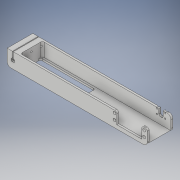
# Autodesk Inventor part: ArmProto1.2
Saved by Autodesk Inventor 2017 (Build 210142000, 142)
## iProperties
Created: 2017-09-30
Part Number: ArmProto1.2
Material: Generic
Document SubType Name: Modeling
Designer: User
Density: 1 g/cm^3
Appearance: Default
Author: User
Autodesk Inventor part; units mm, degrees
ref_plane "YZ Plane" through (0, 0, 0) normal (1, 0, 0) x (0, 1, 0)
ref_plane "XZ Plane" through (0, 0, 0) normal (0, 1, 0) x (-1, 0, 0)
ref_plane "XY Plane" through (0, 0, 0) normal (0, 0, 1) x (1, 0, 0)
sketch "Sketch1" plane through (0, 0, 0) normal (1, 0, 0) x (0, 1, 0)
  line L0 (0, 0) -> (25.4, 0)
  line L1 (25.4, 0) -> (25.4, -42.799)
  line L2 (25.4, -42.799) -> (0, -42.799)
  line L3 (0, -42.799) -> (0, 0)
  line L4 (25.4, -3.175) -> (3.175, -3.175)
  line L5 (3.175, -3.175) -> (3.175, -39.624)
  line L6 (3.175, -39.624) -> (25.4, -39.624)
  line L7 (25.4, -39.624) -> (25.4, -3.175)
  dimension "d0" = 25.4
  dimension "d1" = 42.799
  dimension "d2" = 22.225
  dimension "d3" = 36.449
  dimension "d4" = 3.175
  constraints: 16 end point, 4 parallel, 2 horizontal, 2 perpendicular, 1 point on line
  measures "d0" distance of L1.end L2.end
  measures "d1" distance of L0.end L1.end
  measures "d2" distance of L5.end L6.end
  measures "d3" distance of L4.end L5.end
  measures "d4" distance between parallel lines of L0 L4
extrude "Extrusion1" add sketch "Sketch1" along normal blind 233.6038 contours L0 L1 L4 L5 L6 L2 L3
sketch "Sketch2" plane through (0, 0, 0) normal (0, 0, 1) x (1, 0, 0)
  line L0 (0, 25.4) -> (0, 0) projected
  line L1 (0, 0) -> (233.6038, 0) projected
  line L2 (233.6038, 25.4) -> (233.6038, 0) projected
  line L3 (0, 25.4) -> (233.6038, 25.4) projected
  line L4 (224.7138, 25.4) -> (182.8038, 25.4)
  line L5 (182.8038, 25.4) -> (182.8038, 6.35)
  line L6 (182.8038, 6.35) -> (224.7138, 6.35)
  line L7 (224.7138, 6.35) -> (224.7138, 25.4)
  circle A0 centre (228.6, 21.2344) radius 2.413
  circle A1 centre (228.6, 11.2344) radius 2.413
  circle A2 centre (179.1, 21.2344) radius 2.413
  circle A3 centre (179.1, 11.2344) radius 2.413
  dimension "d7" = 8.89
  dimension "d8" = 25.4
  dimension "d9" = 19.05
  dimension "d10" = 50.8
  dimension "d11" = 4.826
  dimension "d12" = 4.826
  dimension "d13" = 4.1656
  dimension "d14" = 10
  dimension "d15" = 4.826
  dimension "d16" = 4.826
  dimension "d91" = 49.5
  dimension "d92" = 49.5
  dimension "d93" = 4.1656
  dimension "d95" = 10
  dimension "d96" = 5.0038
  dimension "d97" = 5.0038
  constraints: 8 end point, 4 centre point, 2 parallel, 1 horizontal, 1 perpendicular, 1 point on line
  measures "d7" distance between parallel lines of L2 L7
  measures "d8" distance of L2.start L1.end
  measures "d9" distance of L6.end L4.start
  measures "d10" distance between parallel lines of L2 L5
  measures "d11" diameter of A0
  measures "d12" diameter of A1
  measures "d13" distance from line of A0.centre L3
  measures "d14" distance of A1.centre A0.centre
  measures "d15" diameter of A2
  measures "d16" diameter of A3
  measures "d91" distance of A0.centre A2.centre
  measures "d92" distance of A3.centre A1.centre
  measures "d93" distance from line of L3 A2.centre
  measures "d95" distance of A2.centre A3.centre
  measures "d96" distance from line of L2 A0.centre
  measures "d97" distance from line of L2 A1.centre
extrude "Extrusion2" cut sketch "Sketch2" against normal blind 12.7 contours L3 L7 L6 L5 | A0 | A1 | A2 | A3
sketch "Sketch4" plane through (0, 0, 0) normal (0, 0, 1) x (1, 0, 0)
  line L0 (224.7138, 25.4) -> (224.7138, 6.35) projected
  line L1 (224.7138, 6.35) -> (182.8038, 6.35) projected
  line L2 (182.8038, 6.35) -> (182.8038, 25.4) projected
  line L3 (0, 25.4) -> (182.8038, 25.4) projected
  line L4 (0, 25.4) -> (0, 0) projected
  line L5 (0, 0) -> (233.6038, 0) projected
  line L6 (233.6038, 25.4) -> (233.6038, 0) projected
  line L7 (224.7138, 25.4) -> (233.6038, 25.4) projected
  circle A0 centre (179.1, 21.2344) radius 2.413 projected
  circle A1 centre (228.6, 21.2344) radius 2.413 projected
  circle A2 centre (228.6, 11.2344) radius 2.413 projected
  circle A3 centre (179.1, 11.2344) radius 2.413 projected
  line L8 (0, 0) -> (233.6038, 0) projected
  line L9 (19.05, 25.4) -> (19.05, 0)
  line L10 (19.05, 0) -> (0, 0)
  line L11 (0, 0) -> (0, 25.4)
  line L12 (7.8359, 10.2108) -> (11.2141, 10.2108)
  arc A4 (6.8548, 11.3386) -> (7.8359, 10.2108) centre (7.8359, 11.2014) ccw
  arc A5 (11.2141, 10.2108) -> (12.1952, 11.3386) centre (11.2141, 11.2014) ccw
  line L13 (9.525, 10.2108) -> (9.525, 8.4163)
  line L14 (0, 25.4) -> (233.6038, 25.4) projected
  line L15 (10.16, 25.4) -> (10.16, 15.6292)
  line L16 (8.89, 15.6292) -> (8.89, 25.4)
  arc A6 (12.1952, 11.3386) -> (10.16, 15.6292) centre (9.525, 12.7) ccw
  arc A7 (8.89, 15.6292) -> (6.8548, 11.3386) centre (9.525, 12.7) ccw
  line L17 (0, 25.4) -> (8.89, 25.4)
  line L18 (10.16, 25.4) -> (19.05, 25.4)
  dimension "d26" = 19.05
  dimension "d28" = 1.9812
  dimension "d29" = 1.9812
  dimension "d30" = 2.4892
  dimension "d32" = 1.6891
  dimension "d33" = 1.6891
  dimension "d34" = 1.6891
  dimension "d35" = 0
  dimension "d37" = 3.3782
  dimension "d38" = 25.4
  dimension "d39" = 12.7
  dimension "d40" = 9.525
  dimension "d42" = 8.89
  constraints: 18 end point, 8 point on circle, 4 centre point, 4 parallel, 3 horizontal, 3 perpendicular, 2 point on line, 1 coincident, 1 midpoint, 1 tangent
  measures "d26" distance of L9.end L10.end
  measures "d28" diameter of A4
  measures "d29" diameter of A5
  measures "d30" distance from line of L12 point (9.525, 12.7)
  measures "d32" distance from line of L12.start L13
  measures "d33" distance from line of A4.centre L13
  measures "d34" distance from line of A5.centre L13
  measures "d35" distance from line of L13 A6.centre
  measures "d37" distance of L12.start L12.end
  measures "d38" distance of L10.end L3.start
  measures "d39" distance from line of L10 A6.centre
  measures "d40" distance from line of L4 A6.centre
  measures "d42" distance between parallel lines of L4 L16
extrude "Extrusion4" add sketch "Sketch4" against normal blind 42.799 contours L9 L5 L4 L3 L16 A7 A4 L12 A5 A6 L15
sketch "Sketch5" plane through (0, 0, 0) normal (0, 0, 1) x (1, 0, 0)
  line L0 (270.51, 25.4) -> (270.51, 6.35)
  line L1 (270.51, 6.35) -> (228.6, 6.35)
  line L2 (228.6, 6.35) -> (228.6, 25.4)
  line L3 (0, 25.4) -> (10.16, 25.4)
  line L4 (0, 25.4) -> (0, 0)
  line L5 (0, 0) -> (279.4, 0)
  line L6 (279.4, 25.4) -> (279.4, 0)
  line L7 (270.51, 25.4) -> (279.4, 25.4)
  circle A0 centre (225.1202, 21.2344) radius 2.413
  circle A1 centre (274.399, 21.2344) radius 2.413
  circle A2 centre (274.399, 11.2268) radius 2.413
  circle A3 centre (225.1202, 11.2268) radius 2.413
  line L8 (0, 0) -> (279.4, 0)
  line L9 (19.05, 10.2108) -> (19.05, 0)
  line L10 (19.05, 0) -> (0, 0)
  line L11 (0, 0) -> (0, 25.4)
  line L12 (7.8359, 10.2108) -> (11.2141, 10.2108)
  arc A4 (6.8548, 11.3386) -> (7.8359, 10.2108) centre (7.8359, 11.2014) ccw
  arc A5 (11.2141, 10.2108) -> (12.1952, 11.3386) centre (11.2141, 11.2014) ccw
  line L13 (9.525, 10.2108) -> (9.525, 8.4163)
  line L14 (10.16, 25.4) -> (10.16, 15.6292)
  line L15 (8.89, 15.6292) -> (8.89, 25.4)
  arc A6 (12.1952, 11.3386) -> (10.16, 15.6292) centre (9.525, 12.7) ccw
  arc A7 (8.89, 15.6292) -> (6.8548, 11.3386) centre (9.525, 12.7) ccw
  line L16 (0, 25.4) -> (8.89, 25.4)
  line L17 (0, 25.4) -> (10.16, 25.4)
  line L18 (228.6, 25.4) -> (279.4, 25.4)
  dimension "d45" = 19.05
  dimension "d46" = 1.9812
  dimension "d47" = 1.9812
  dimension "d48" = 2.4892
  dimension "d49" = 1.6891
  dimension "d50" = 1.6891
  dimension "d51" = 1.6891
  dimension "d52" = 0
  dimension "d53" = 3.3782
  dimension "d54" = 25.4
  dimension "d55" = 12.7
  dimension "d56" = 9.525
  dimension "d57" = 8.89
  constraints: 38 end point, 8 centre point, 8 point on circle, 3 parallel, 3 point on line, 2 horizontal, 2 perpendicular, 1 coincident, 1 midpoint, 1 tangent
  measures "d45" distance of L9.end L10.end
  measures "d46" diameter of A4
  measures "d47" diameter of A5
  measures "d48" distance from line of L12 point (9.525, 12.7)
  measures "d49" distance from line of L12.start L13
  measures "d50" distance from line of A4.centre L13
  measures "d51" distance from line of A5.centre L13
  measures "d52" distance from line of L13 A6.centre
  measures "d53" distance of L12.start L12.end
  measures "d54" distance of L10.end L3.start
  measures "d55" distance from line of L10 A6.centre
  measures "d56" distance from line of L4 A6.centre
  measures "d57" distance between parallel lines of L4 L15
extrude "Extrusion5" cut sketch "Sketch5" against normal blind 42.799 contours L3 L14 A6 A5 L12 A4 A7 L15
sketch "Sketch6" plane through (0, 0, 0) normal (-1, 0, 0) x (0, 0, 1)
  line L0 (-42.799, 25.4) -> (0, 25.4) projected
  line L1 (-42.799, 0) -> (-42.799, 25.4) projected
  line L2 (0, 0) -> (-42.799, 0) projected
  line L3 (0, 25.4) -> (0, 0) projected
  point P0 (-37.4491, 19.05)
  point P1 (-5.3499, 19.05)
  point P2 (-21.3995, 19.05)
  dimension "d62" = 6.35
  dimension "d63" = 6.35
  dimension "d64" = 42.799
  dimension "d65" = 6.35
  dimension "d66" = 21.3995
  dimension "d67" = 5.3499
  dimension "d68" = 5.3499
  measures "d62" distance from line of L0 point (-5.35, 19.05)
  measures "d63" distance from line of L0 point (-37.449, 19.05)
  measures "d64" distance of L0.start L0.end
  measures "d65" distance from line of L0 point (-21.4, 19.05)
  measures "d66" distance from line of L3 point (-21.4, 19.05)
  measures "d67" distance from line of L3 point (-5.35, 19.05)
  measures "d68" distance from line of L1 point (-37.449, 19.05)
hole "Hole1" at (0, 19.05, -37.4491) at (0, 19.05, -5.3499) at (0, 19.05, -21.3995) direction (1, 0, 0) diameter 4.0132 depth 9.017 tip angle 118
sketch "Sketch7" plane through (10.16, 15.6292, 0) normal (-1, 0, 0) x (0, 0, 1)
  circle A0 centre (-5.3499, 3.4208) radius 2.0066 projected
  circle A1 centre (-37.4491, 3.4208) radius 2.0066 projected
  circle A2 centre (-21.3995, 3.4208) radius 2.0066 projected
  line L0 (-42.799, 9.7708) -> (0, 9.7708) projected
  line L1 (-42.799, -15.6292) -> (-42.799, 9.7708) projected
  line L2 (0, -15.6292) -> (-42.799, -15.6292) projected
  line L3 (0, 9.7708) -> (0, -15.6292) projected
hole "Hole2" at (10.16, 19.05, -37.4491) at (10.16, 19.05, -21.3995) at (10.16, 19.05, -5.3499) direction (1, 0, 0) diameter 2.6416 end through all thread size "6-32 UNC" class "2B" standard "ANSI Unified Screw Threads"
fillet "Fillet1" radius 3.175 2 edges at (19.05, 14.2875, -39.624) (19.05, 14.2875, -3.175)
fillet "Fillet2" radius 6.35 3 edges at (0, 0, -21.3995) (233.6038, 25.4, -41.2115) (233.6038, 0, -21.3995)
fillet "Fillet3" radius 3.175 3 edges at (233.6038, 25.4, -1.5875) (182.8038, 25.4, -1.5875) (224.7138, 25.4, -1.5875)
sketch "Sketch9" plane through (6.35, 0, 0) normal (0, -1, 0) x (1, 0, 0)
  line L0 (220.9038, 0) -> (220.9038, -42.799) projected
  line L1 (0, 0) -> (220.9038, 0) projected
  line L2 (0, -42.799) -> (0, 0) projected
  line L3 (0, -42.799) -> (220.9038, -42.799) projected
  line L4 (12.7, -36.449) -> (104.1019, -36.449)
  line L5 (104.1019, -36.449) -> (104.1019, -6.35)
  line L6 (104.1019, -6.35) -> (12.7, -6.35)
  line L7 (12.7, -6.35) -> (12.7, -36.449)
  point P0 (-6.35, 0)
  dimension "d107" = 42.799
  dimension "d108" = 220.9038
  dimension "d109" = 12.7
  dimension "d110" = 6.35
  dimension "d111" = 30.099
  dimension "d112" = 91.4019
  constraints: 8 end point, 2 parallel, 1 horizontal, 1 perpendicular
  measures "d107" distance of L2.start L1.start
  measures "d108" distance of L1.start L0.start
  measures "d109" distance between parallel lines of L2 L7
  measures "d110" distance between parallel lines of L1 L6
  measures "d111" distance of L6.end L4.start
  measures "d112" distance of L5.end L6.end
extrude "Extrusion6" cut sketch "Sketch9" against normal blind 25.4 contours L7 L6 L5 L4
fillet "Fillet4" radius 3.175 4 edges at (19.05, 1.5875, -6.35) (19.05, 1.5875, -36.449) (110.4519, 1.5875, -6.35) (110.4519, 1.5875, -36.449)
sketch "Sketch10" plane through (8.89, 25.4, -42.799) normal (0, 0, -1) x (-1, 0, 0)
  arc A0 (-224.7138, -19.05) -> (-218.3638, -25.4) centre (-218.3638, -19.05) ccw projected
  line L0 (2.54, -25.4) -> (-218.3638, -25.4) projected
  arc A1 (2.54, -25.4) -> (8.89, -19.05) centre (2.54, -19.05) ccw projected
  line L1 (8.89, -19.05) -> (8.89, 0) projected
  line L2 (8.89, 0) -> (0, 0) projected
  line L3 (0, 0) -> (0, -9.7708) projected
  arc A2 (2.0352, -14.0614) -> (0, -9.7708) centre (-0.635, -12.7) ccw projected
  arc A3 (1.0541, -15.1892) -> (2.0352, -14.0614) centre (1.0541, -14.1986) ccw projected
  line L4 (1.0541, -15.1892) -> (-2.3241, -15.1892) projected
  arc A4 (-3.3052, -14.0614) -> (-2.3241, -15.1892) centre (-2.3241, -14.1986) ccw projected
  arc A5 (-1.27, -9.7708) -> (-3.3052, -14.0614) centre (-0.635, -12.7) ccw projected
  line L5 (-1.27, -9.7708) -> (-1.27, 0) projected
  line L6 (-1.27, 0) -> (-218.3638, 0) projected
  arc A6 (-218.3638, 0) -> (-224.7138, -6.35) centre (-218.3638, -6.35) ccw projected
  line L7 (-224.7138, -19.05) -> (-224.7138, -6.35) projected
  line L8 (-211.7292, 0) -> (-204.7292, 0)
  line L9 (-204.7292, 0) -> (-204.7292, -10.7404)
  line L10 (-204.7292, -10.7404) -> (-211.7292, -10.7404)
  line L11 (-211.7292, -10.7404) -> (-211.7292, 0)
  circle A7 centre (-215.1634, -9.6266) radius 1.23
  circle A8 centre (-201.2956, -9.7536) radius 1.23
  circle A9 centre (-215.1634, -1.6256) radius 1.23
  circle A10 centre (-201.295, -1.6256) radius 1.23
  point P0 (8.89, -25.4)
  dimension "d122" = 13.8684
  dimension "d125" = 7
  dimension "d126" = 25.4
  dimension "d127" = 10.7404
  dimension "d128" = 2.46
  dimension "d129" = 2.46
  dimension "d130" = 0
  dimension "d131" = 15.7734
  dimension "d132" = 9.5504
  dimension "d135" = 3.4342
  dimension "d136" = 2.46
  dimension "d137" = 2.46
  dimension "d138" = 9.5504
  dimension "d139" = 23.7744
  dimension "d140" = 23.7744
  constraints: 8 end point, 4 centre point, 2 coincident, 2 parallel, 1 horizontal, 1 perpendicular
  measures "d122" distance of point (-215.163, -9.627) point (-201.296, -9.754)
  measures "d125" distance of L8.start L8.end
  measures "d126" distance between parallel lines of L0 L6
  measures "d127" distance of L8.end L9.end
  measures "d128" diameter of A7
  measures "d129" diameter of A8
  measures "d130" distance between parallel lines of L6 L8
  measures "d131" distance from line of L0 A7.centre
  measures "d132" distance from line of L7 A7.centre
  measures "d135" distance from line of A7.centre L11
  measures "d136" diameter of A9
  measures "d137" diameter of A10
  measures "d138" distance from line of L7 A9.centre
  measures "d139" distance from line of L0 A9.centre
  measures "d140" distance from line of L0 A10.centre
extrude "Extrusion7" cut sketch "Sketch10" against normal blind 6.35 contours L6 L9 L10 L11 | A7 | A8 | A9 | A10
fillet "Fillet5" radius 2.54 2 edges at (213.6192, 14.6596, -41.2115) (220.6192, 14.6596, -41.2115)
sketch "Sketch11" plane through (8.89, 25.4, -42.799) normal (0, 0, -1) x (-1, 0, 0)
  line L0 (-211.7292, -8.2004) -> (-211.7292, 0) projected
  line L1 (-211.7292, 0) -> (-218.3638, 0) projected
  arc A0 (-218.3638, 0) -> (-224.7138, -6.35) centre (-218.3638, -6.35) ccw projected
  line L2 (-224.7138, -19.05) -> (-224.7138, -6.35) projected
  arc A1 (-224.7138, -19.05) -> (-218.3638, -25.4) centre (-218.3638, -19.05) ccw projected
  line L3 (2.54, -25.4) -> (-218.3638, -25.4) projected
  arc A2 (2.54, -25.4) -> (8.89, -19.05) centre (2.54, -19.05) ccw projected
  line L4 (8.89, -19.05) -> (8.89, 0) projected
  line L5 (8.89, 0) -> (0, 0) projected
  line L6 (0, 0) -> (0, -9.7708) projected
  arc A3 (2.0352, -14.0614) -> (0, -9.7708) centre (-0.635, -12.7) ccw projected
  arc A4 (1.0541, -15.1892) -> (2.0352, -14.0614) centre (1.0541, -14.1986) ccw projected
  line L7 (1.0541, -15.1892) -> (-2.3241, -15.1892) projected
  arc A5 (-3.3052, -14.0614) -> (-2.3241, -15.1892) centre (-2.3241, -14.1986) ccw projected
  arc A6 (-1.27, -9.7708) -> (-3.3052, -14.0614) centre (-0.635, -12.7) ccw projected
  line L8 (-1.27, -9.7708) -> (-1.27, 0) projected
  line L9 (-1.27, 0) -> (-204.7292, 0) projected
  line L10 (-204.7292, 0) -> (-204.7292, -8.2004) projected
  arc A7 (-207.2692, -10.7404) -> (-204.7292, -8.2004) centre (-207.2692, -8.2004) ccw projected
  line L11 (-207.2692, -10.7404) -> (-209.1892, -10.7404) projected
  arc A8 (-211.7292, -8.2004) -> (-209.1892, -10.7404) centre (-209.1892, -8.2004) ccw projected
  circle A9 centre (-201.295, -1.6256) radius 1.23 projected
  circle A10 centre (-201.2956, -9.7536) radius 1.23 projected
  circle A11 centre (-215.1634, -9.6266) radius 1.23 projected
  circle A12 centre (-215.1634, -1.6256) radius 1.23 projected
  circle A13 centre (-215.1634, -9.6266) radius 1.23 projected
  point P0 (8.89, -25.4)
  constraints: 4 coincident
hole "Hole5" at (210.185, 23.7744, -42.799) at (210.1856, 15.6464, -42.799) at (224.0534, 23.7744, -42.799) at (224.0534, 15.7734, -42.799) direction (0, 0, 1) diameter 2.4638 depth 25.4 tip angle 118 countersink diameter 6 countersink angle 90
equation "\"d12\" = d11"
equation "\"d15\" = d11"
equation "\"d16\" = d11"
equation "\"d92\" = d91"
equation "\"d93\" = d13"
equation "\"d95\" = d14"
equation "\"d97\" = d96"
equation "\"d29\" = d28"
equation "\"d32\" = 0.5 * d27"
equation "\"d33\" = d32"
equation "\"d34\" = d32"
equation "\"d39\" = 0.5 * d38"
equation "\"d40\" = 0.5 * d26"
equation "\"d42\" = 0.5 * d26 - 0.5 * d41"
equation "\"d47\" = d46"
equation "\"d49\" = 0.5 * d58"
equation "\"d50\" = d49"
equation "\"d51\" = d49"
equation "\"d55\" = 0.5 * d54"
equation "\"d56\" = 0.5 * d45"
equation "\"d57\" = 0.5 * d45 - 0.5 * d59"
equation "\"d63\" = d62"
equation "\"d65\" = d62"
equation "\"d66\" = 0.5 * d64"
equation "\"d67\" = 0.125 * d64"
equation "\"d68\" = d67"
equation "\"d128\" = d129"
equation "\"d135\" = -0.5 * d125 + 0.5 * d122"
equation "\"d136\" = d129"
equation "\"d137\" = d129"
equation "\"d138\" = d132"
equation "\"d140\" = d139"
equation "\"d27\" = 3.3782"
equation "\"d41\" = 1.27"
equation "\"d58\" = 3.3782"
equation "\"d59\" = 1.27"
body "Solid1"
